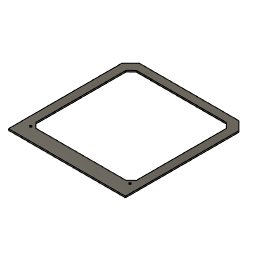
cvqa_camera_mount_assy v8 (Autodesk Fusion 360 archive; units mm, degrees)
design "varian_tray"
Autodesk Fusion 360 part; units mm, degrees
sketch "Sketch1" plane through (0, 0, 0) normal (0, 0, 1) x (1, 0, 0)
  line L0 (135, 141) -> (-135, 141)
  line L1 (-135, 141) -> (-135, -141)
  line L2 (-135, -141) -> (135, -141)
  line L3 (135, -141) -> (135, 141)
  line L4 (135, 141) -> (-135, -141) construction
  line L5 (-135, 141) -> (135, -141) construction
  line L6 (-104.0059, 123) -> (104.0059, 123)
  line L7 (104, -108.6222) -> (-104, -108.6222)
  line L8 (-116, 111.3778) -> (-104.0059, 123)
  line L9 (-116, -96.6222) -> (-116, 111.3778)
  line L10 (-116, 121.1556) -> (-116, 123.3778)
  line L11 (0, 86.9957) -> (0, -79.0579) construction
  line L12 (116, 111.3778) -> (104.0059, 123)
  line L13 (116, 123.3776) -> (116, 121.1556)
  line L14 (116, 111.3778) -> (116, -96.6222)
  line L15 (-116, -96.6222) -> (-104, -108.6222)
  line L16 (104, -108.6222) -> (116, -96.6222)
  circle A0 centre (-114.5, -110) radius 2.2479
  circle A1 centre (114.5, -110) radius 2.2479
  dimension "d1" = 270
  dimension "d2" = 282
  dimension "d3" = 232
  dimension "d5" = 18
  dimension "d6" = 19
  dimension "d7" = 12
  dimension "d8" = 12
  dimension "d13" = 4.4958
  dimension "d14" = 4.4958
  dimension "d15" = 229
  dimension "d16" = 31
  dimension "d17" = 20.5
  constraint horizontal L0
  constraint perpendicular L0 L1
  constraint parallel L0 L2
  constraint parallel L1 L3
  constraint coincident L4 origin
  constraint coincident L5 origin
  constraint horizontal L6
  constraint vertical L13
  constraint horizontal L7
  constraint vertical L9
  constraint coincident L8.start L9.end
  constraint coincident L6.start L8.end
  constraint coincident L5 L10.start
  constraint collinear L9 L10
  constraint vertical L11
  constraint symmetric L8.start L11 L12.start
  constraint symmetric L6.start L11 L6.end
  constraint coincident L4 L13.end
  constraint collinear L13 L14
  constraint coincident L4 L7.end
  constraint coincident L9.start L15.start
  constraint coincident L7.end L15.end
  constraint coincident L7.start L16.start
  constraint coincident L14.end L16.end
  measures "d1" distance of L1.end L2.end
  measures "d2" distance of L0.end L1.end
  measures "d3" distance of L10.end L13.start
  measures "d5" distance of L0 L6
  measures "d6" distance of L1 L9
  measures "d7" distance of L10.end L6.start
  measures "d8" distance of L10.end L8.start
  measures "d13" diameter of A0
  measures "d14" diameter of A1
  measures "d15" distance of A0.centre A1.centre
  measures "d16" distance of L2 A1.centre
  measures "d17" distance of L1 A0.centre
extrude "Extrude1" add sketch "Sketch1" along normal blind 3.1
chamfer "Chamfer1" distance 20 angle 45 2 edges at (135, 141, 1.55) (-135, 141, 1.55)
chamfer "Chamfer2" distance 2.286 angle 45 2 edges at (112.4042, -109.1871, 0) (-116.5958, -109.1871, 0)
equation "d6 = ( ( 270 - 232 ) / 2 ) * 1 mm"
equation "d17 = ( ( 270 - 229 ) / 2 ) * 1 mm"
